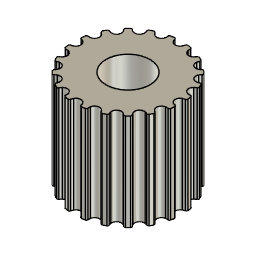
PC_v1 (Autodesk Fusion 360 design; units mm, degrees)
part number: 2026-03-17-17-27-52-163
Autodesk Fusion 360 part; units mm, degrees
sketch "Pulley" plane through (0, 0, 0) normal (0, 0, 1) x (-1, 0, 0)
  circle A0 centre (-25, -15) radius 6.1122
  line L0 (-25, -15) -> (-25, -21.1122)
  line L1 (-25, -21.1122) -> (-25, -20.9172)
  line L2 (-25, -15) -> (-31.1122, -15) construction
  line L3 (-25, -15) -> (-18.8878, -15) construction
  line L4 (-25, -21.1122) -> (-24.6, -21.1122)
  line L5 (-25, -21.1122) -> (-25.4, -21.1122)
  circle A1 centre (-25, -15) radius 2.5
  arc A2 (-24.5011, -20.674) -> (-25.4989, -20.674) centre (-25, -20.9172) ccw
  arc A3 (-25.4989, -20.674) -> (-25.5996, -21.0827) centre (-24.6, -21.1122) ccw
  arc A4 (-24.4004, -21.0827) -> (-24.5011, -20.674) centre (-25.4, -21.1122) ccw
  line L6 (-25.7517, -21.0658) -> (-25.7517, -21.0658)
  arc A5 (-24.4145, -20.9424) -> (-24.2483, -21.0658) centre (-24.2667, -20.9169) ccw
  arc A6 (-25.7517, -21.0658) -> (-25.5855, -20.9424) centre (-25.7333, -20.9169) ccw
  arc A7 (-23.8405, -21.0012) -> (-23.7205, -20.8325) centre (-23.869, -20.8539) ccw
  arc A8 (-23.7211, -20.5505) -> (-23.6906, -20.9703) centre (-22.7308, -20.6894) ccw
  arc A9 (-22.7722, -20.2422) -> (-23.7211, -20.5505) centre (-23.1715, -20.6276) ccw
  arc A10 (-22.5501, -20.5997) -> (-22.7722, -20.2422) centre (-23.4917, -20.9367) ccw
  arc A11 (-22.6069, -20.4706) -> (-22.4106, -20.5366) centre (-22.4742, -20.4007) ccw
  arc A12 (-22.0428, -20.3492) -> (-21.9808, -20.1516) centre (-22.1154, -20.2179) ccw
  arc A13 (-22.0685, -19.8836) -> (-21.9097, -20.2734) centre (-21.0837, -19.7098) ccw
  arc A14 (-21.2613, -19.2971) -> (-22.0685, -19.8836) centre (-21.522, -19.7871) ccw
  arc A15 (-20.9396, -19.5686) -> (-21.2613, -19.2971) centre (-21.7309, -20.18) ccw
  arc A16 (-21.0335, -19.4634) -> (-20.8264, -19.4655) centre (-20.9289, -19.3559) ccw
  arc A17 (-20.5345, -19.1736) -> (-20.5366, -18.9665) centre (-20.6441, -19.0711) ccw
  arc A18 (-20.7029, -18.7387) -> (-20.4314, -19.0604) centre (-19.82, -18.2691) ccw
  arc A19 (-20.1164, -17.9315) -> (-20.7029, -18.7387) centre (-20.2129, -18.478) ccw
  arc A20 (-19.7266, -18.0903) -> (-20.1164, -17.9315) centre (-20.2902, -18.9163) ccw
  arc A21 (-19.8484, -18.0192) -> (-19.6508, -17.9572) centre (-19.7821, -17.8846) ccw
  arc A22 (-19.4634, -17.5894) -> (-19.5294, -17.3931) centre (-19.5993, -17.5258) ccw
  arc A23 (-19.7578, -17.2279) -> (-19.4003, -17.4499) centre (-19.0633, -16.5084) ccw
  arc A24 (-19.4495, -16.2789) -> (-19.7578, -17.2279) centre (-19.3724, -16.8285) ccw
  arc A25 (-19.0297, -16.3094) -> (-19.4495, -16.2789) centre (-19.3106, -17.2692) ccw
  arc A26 (-19.1675, -16.2795) -> (-18.9988, -16.1595) centre (-19.1461, -16.131) ccw
  arc A27 (-18.9342, -15.7517) -> (-19.0576, -15.5855) centre (-19.0831, -15.7333) ccw
  arc A28 (-19.326, -15.4989) -> (-18.9173, -15.5996) centre (-18.8878, -14.6) ccw
  arc A29 (-19.326, -14.5011) -> (-19.326, -15.4989) centre (-19.0828, -15) ccw
  arc A30 (-18.9173, -14.4004) -> (-19.326, -14.5011) centre (-18.8878, -15.4) ccw
  arc A31 (-19.0576, -14.4145) -> (-18.9342, -14.2483) centre (-19.0831, -14.2667) ccw
  arc A32 (-18.9988, -13.8405) -> (-19.1675, -13.7205) centre (-19.1461, -13.869) ccw
  arc A33 (-19.4495, -13.7211) -> (-19.0297, -13.6906) centre (-19.3106, -12.7308) ccw
  arc A34 (-19.7578, -12.7722) -> (-19.4495, -13.7211) centre (-19.3724, -13.1715) ccw
  arc A35 (-19.4003, -12.5501) -> (-19.7578, -12.7722) centre (-19.0633, -13.4916) ccw
  arc A36 (-19.5294, -12.6069) -> (-19.4634, -12.4106) centre (-19.5993, -12.4742) ccw
  arc A37 (-19.6508, -12.0428) -> (-19.8484, -11.9808) centre (-19.7821, -12.1154) ccw
  arc A38 (-20.1164, -12.0685) -> (-19.7266, -11.9097) centre (-20.2902, -11.0837) ccw
  arc A39 (-20.7029, -11.2613) -> (-20.1164, -12.0685) centre (-20.2129, -11.522) ccw
  arc A40 (-20.4314, -10.9396) -> (-20.7029, -11.2613) centre (-19.82, -11.7309) ccw
  arc A41 (-20.5366, -11.0335) -> (-20.5345, -10.8264) centre (-20.6441, -10.9289) ccw
  arc A42 (-20.8264, -10.5345) -> (-21.0335, -10.5366) centre (-20.9289, -10.6441) ccw
  arc A43 (-21.2613, -10.7029) -> (-20.9396, -10.4314) centre (-21.7309, -9.82) ccw
  arc A44 (-22.0685, -10.1164) -> (-21.2613, -10.7029) centre (-21.522, -10.2129) ccw
  arc A45 (-21.9097, -9.7266) -> (-22.0685, -10.1164) centre (-21.0837, -10.2902) ccw
  arc A46 (-21.9808, -9.8484) -> (-22.0428, -9.6508) centre (-22.1154, -9.7821) ccw
  arc A47 (-22.4106, -9.4634) -> (-22.6069, -9.5294) centre (-22.4742, -9.5993) ccw
  arc A48 (-22.7721, -9.7578) -> (-22.5501, -9.4003) centre (-23.4917, -9.0633) ccw
  arc A49 (-23.7211, -9.4495) -> (-22.7721, -9.7578) centre (-23.1715, -9.3724) ccw
  arc A50 (-23.6906, -9.0297) -> (-23.7211, -9.4495) centre (-22.7308, -9.3106) ccw
  arc A51 (-23.7205, -9.1675) -> (-23.8405, -8.9988) centre (-23.869, -9.1461) ccw
  arc A52 (-24.2483, -8.9342) -> (-24.4145, -9.0576) centre (-24.2667, -9.0831) ccw
  arc A53 (-24.5011, -9.326) -> (-24.4004, -8.9173) centre (-25.4, -8.8878) ccw
  arc A54 (-25.4989, -9.326) -> (-24.5011, -9.326) centre (-25, -9.0828) ccw
  arc A55 (-25.5996, -8.9173) -> (-25.4989, -9.326) centre (-24.6, -8.8878) ccw
  arc A56 (-25.5855, -9.0576) -> (-25.7518, -8.9342) centre (-25.7333, -9.0831) ccw
  arc A57 (-26.1595, -8.9988) -> (-26.2795, -9.1675) centre (-26.131, -9.1461) ccw
  arc A58 (-26.2789, -9.4495) -> (-26.3094, -9.0297) centre (-27.2692, -9.3106) ccw
  arc A59 (-27.2278, -9.7578) -> (-26.2789, -9.4495) centre (-26.8285, -9.3724) ccw
  arc A60 (-27.4499, -9.4003) -> (-27.2278, -9.7578) centre (-26.5084, -9.0633) ccw
  arc A61 (-27.3931, -9.5294) -> (-27.5894, -9.4634) centre (-27.5258, -9.5993) ccw
  arc A62 (-27.9572, -9.6508) -> (-28.0192, -9.8484) centre (-27.8846, -9.7821) ccw
  arc A63 (-27.9315, -10.1164) -> (-28.0903, -9.7266) centre (-28.9163, -10.2902) ccw
  arc A64 (-28.7387, -10.7029) -> (-27.9315, -10.1164) centre (-28.478, -10.2129) ccw
  arc A65 (-29.0604, -10.4314) -> (-28.7387, -10.7029) centre (-28.2691, -9.82) ccw
  arc A66 (-28.9665, -10.5366) -> (-29.1736, -10.5345) centre (-29.0711, -10.6441) ccw
  arc A67 (-29.4655, -10.8264) -> (-29.4634, -11.0335) centre (-29.3559, -10.9289) ccw
  arc A68 (-29.2971, -11.2613) -> (-29.5686, -10.9396) centre (-30.18, -11.7309) ccw
  arc A69 (-29.8836, -12.0685) -> (-29.2971, -11.2613) centre (-29.7871, -11.522) ccw
  arc A70 (-30.2734, -11.9097) -> (-29.8836, -12.0685) centre (-29.7098, -11.0837) ccw
  arc A71 (-30.1516, -11.9808) -> (-30.3492, -12.0428) centre (-30.2179, -12.1154) ccw
  arc A72 (-30.5366, -12.4106) -> (-30.4706, -12.6069) centre (-30.4007, -12.4742) ccw
  arc A73 (-30.2422, -12.7721) -> (-30.5997, -12.5501) centre (-30.9367, -13.4916) ccw
  arc A74 (-30.5505, -13.7211) -> (-30.2422, -12.7721) centre (-30.6276, -13.1715) ccw
  arc A75 (-30.9703, -13.6906) -> (-30.5505, -13.7211) centre (-30.6894, -12.7308) ccw
  arc A76 (-30.8325, -13.7205) -> (-31.0012, -13.8405) centre (-30.8539, -13.869) ccw
  arc A77 (-31.0658, -14.2483) -> (-30.9424, -14.4145) centre (-30.9169, -14.2667) ccw
  arc A78 (-30.674, -14.5011) -> (-31.0827, -14.4004) centre (-31.1122, -15.4) ccw
  arc A79 (-30.674, -15.4989) -> (-30.674, -14.5011) centre (-30.9172, -15) ccw
  arc A80 (-31.0827, -15.5996) -> (-30.674, -15.4989) centre (-31.1122, -14.6) ccw
  arc A81 (-30.9424, -15.5855) -> (-31.0658, -15.7517) centre (-30.9169, -15.7333) ccw
  arc A82 (-31.0012, -16.1595) -> (-30.8325, -16.2795) centre (-30.8539, -16.131) ccw
  arc A83 (-30.5505, -16.2789) -> (-30.9703, -16.3094) centre (-30.6894, -17.2692) ccw
  arc A84 (-30.2422, -17.2278) -> (-30.5505, -16.2789) centre (-30.6276, -16.8285) ccw
  arc A85 (-30.5997, -17.4499) -> (-30.2422, -17.2278) centre (-30.9367, -16.5084) ccw
  arc A86 (-30.4706, -17.3931) -> (-30.5366, -17.5894) centre (-30.4007, -17.5258) ccw
  arc A87 (-30.3492, -17.9572) -> (-30.1516, -18.0192) centre (-30.2179, -17.8846) ccw
  arc A88 (-29.8836, -17.9315) -> (-30.2734, -18.0903) centre (-29.7098, -18.9163) ccw
  arc A89 (-29.2971, -18.7387) -> (-29.8836, -17.9315) centre (-29.7871, -18.478) ccw
  arc A90 (-29.5686, -19.0604) -> (-29.2971, -18.7387) centre (-30.18, -18.2691) ccw
  arc A91 (-29.4634, -18.9665) -> (-29.4655, -19.1736) centre (-29.3559, -19.0711) ccw
  arc A92 (-29.1736, -19.4655) -> (-28.9665, -19.4634) centre (-29.0711, -19.3559) ccw
  arc A93 (-28.7387, -19.2971) -> (-29.0604, -19.5686) centre (-28.2691, -20.18) ccw
  arc A94 (-27.9315, -19.8836) -> (-28.7387, -19.2971) centre (-28.478, -19.7871) ccw
  arc A95 (-28.0903, -20.2734) -> (-27.9315, -19.8836) centre (-28.9163, -19.7098) ccw
  arc A96 (-28.0192, -20.1516) -> (-27.9572, -20.3492) centre (-27.8846, -20.2179) ccw
  arc A97 (-27.5894, -20.5366) -> (-27.3931, -20.4706) centre (-27.5258, -20.4007) ccw
  arc A98 (-27.2279, -20.2422) -> (-27.4499, -20.5997) centre (-26.5084, -20.9367) ccw
  arc A99 (-26.2789, -20.5505) -> (-27.2279, -20.2422) centre (-26.8285, -20.6276) ccw
  arc A100 (-26.3094, -20.9703) -> (-26.2789, -20.5505) centre (-27.2692, -20.6894) ccw
  arc A101 (-26.2795, -20.8325) -> (-26.1595, -21.0012) centre (-26.131, -20.8539) ccw
  point P0 (-24.737, -21.1065)
  point P1 (-25.2471, -21.1072)
  dimension "d17" = 12.2244
  dimension "d18" = 6.1122
  dimension "d20" = 0.195
  dimension "d28" = 0.4
  dimension "d29" = 0.4
  dimension "d44" = 5
  dimension "d61" = 0.555
  dimension "d62" = 2
  dimension "d63" = 2
  dimension "d64" = 0.15
  dimension "d65" = 0.15
  dimension "d67" = 360
  constraint coincident A0.centre L0.start
  constraint vertical L0
  constraint parallel L0 L1
  constraint horizontal L2
  constraint horizontal L3
  constraint perpendicular L1 L4
  constraint perpendicular L0 L5
  constraint coincident A0 P0
  constraint coincident A0 P1
  constraint coincident L1.end A2.centre
  constraint coincident L4.end A3.centre
  constraint coincident L5.end A4.centre
  constraint coincident A0 A3.end
  constraint coincident A0 A4.start
  constraint tangent A0 L6
  constraint tangent L6 A6
  constraint tangent A4 A5
  constraint tangent A0 A5
  constraint tangent A3 A6
  constraint tangent A0 A6
  constraint coincident A3 A6.end
  constraint coincident A4 A5.start
  constraint coincident A0 A5.end
  measures "d17" diameter of A0
  measures "d18" distance of A0.centre L0.end
  measures "d20" distance of L0.end L1.end
  measures "d28" distance of L0.end L4.end
  measures "d29" distance of L0.end L5.end
  measures "d44" diameter of A1
  measures "d61" radius of A2
  measures "d62" diameter of A3
  measures "d63" diameter of A4
  measures "d64" radius of A5
  measures "d65" radius of A6
extrude "Extrude3" add sketch "Pulley" along normal blind 11 contours A0 A2 A3 A4 A5 A6 A7 A8 A9 A10 A11 A12 A13 A14 A15 A16 A17 A18 A19 A20 A21 A22 A23 A24 A25 A26 A27 A28 A29 A30 A31 A32 A33 A34 A35 A36 A37 A38 A39 A40 A41 A42 A43 A44 A45 A46 A47 A48 A49 A50 A51 A52 A53 A54 A55 A56 A57 A58 A59 A60 A61 A62 A63 A64 A65 A66 A67 A68 A69 A70 A71 A72 A73 A74 A75 A76 A77 A78 A79 A80 A81 A82 A83 A84 A85 A86 A87 A88 A89 A90 A91 A92 A93 A94 A95 A96 A97 A98 A99 A100 A101
equation "d17 = ( pd ) * 1 mm"
equation "d18 = ( ( pd / 2 mm ) * 1 mm ) * 1 mm"
equation "d20 = 0.75 mm - ( 0.555 ) * 1 mm"
equation "pd = ( bt * 2 / ( PI ) ) - ( 0.254 * 2 )"
equation "teeth = 20" comment "Enter # of teeth on pulley Note: When changing the # of teeth, if teeth are missing edit the extrude, remove all selections, then select the correct area."
equation "d41 = pw"
equation "bore = 5 mm" comment "Enter bore diameter"
equation "d44 = pb"
equation "pw = if(beltwidth == 9 mm; 11 mm; if(beltwidth == 10 mm; 11 mm; beltwidth + 1 mm))"
equation "d66 = bt"
equation "beltwidth = 9 mm" comment "Enter belt width"
equation "pb = if(bore >= ( ( pd ) * 1 mm - 2 mm ); 5 mm; bore)"
equation "bt = if(teeth < 16; 16; teeth)"
